Top Bearing Cover_v1 (Autodesk Fusion 360 design; units mm, degrees)
Autodesk Fusion 360 part; units mm, degrees
sketch "Sketch1" plane through (0, 0, 0) normal (1, 0, 0) x (0, 1, 0)
  line L0 (0, 0) -> (15, 0) construction
  line L1 (15, 0) -> (15, 4.5) construction
  circle A0 centre (15, 4.5) radius 3
  line L2 (15, 0) -> (11, 0) construction
  line L3 (11, 0) -> (19, 0)
  line L4 (19, 0) -> (19, 3.75)
  line L5 (19, 3.75) -> (11, 3.75)
  line L6 (11, 3.75) -> (2.8, 3.75)
  line L7 (2.8, 3.75) -> (2.8, 0)
  line L8 (2.8, 0) -> (11, 0)
  dimension "d1" = 15
  dimension "d2" = 4.5
  dimension "d3" = 6
  dimension "d4" = 4
  dimension "d5" = 8
  dimension "d6" = 3.75
  dimension "d7" = 2.8
  constraint coincident L0.start origin
  constraint horizontal L0
  constraint perpendicular L0 L1
  constraint coincident L1.end A0.centre
  constraint perpendicular L1 L2
  constraint horizontal L3
  constraint vertical L4
  constraint horizontal L5
  constraint horizontal L6
  constraint vertical L7
  constraint horizontal L8
  constraint coincident L0 L7.end
  measures "d1" distance of L0.start L0.end
  measures "d2" distance of L0.end L1.end
  measures "d3" diameter of A0
  measures "d4" distance of L0.end L2.end
  measures "d5" distance of L2.end L3.end
  measures "d6" distance of L2.end L5.end
  measures "d7" distance of L0.start L7
revolve "Revolve1" add sketch "Sketch1" angle 360 about axis through (0, 0, 1.75) along (0, 0, 1) contours A0 L3 L4 L5 L6 L7 L8
fillet "Fillet1" radius 1.5 1 edges at (-17.7142, 6.8707, 0)
